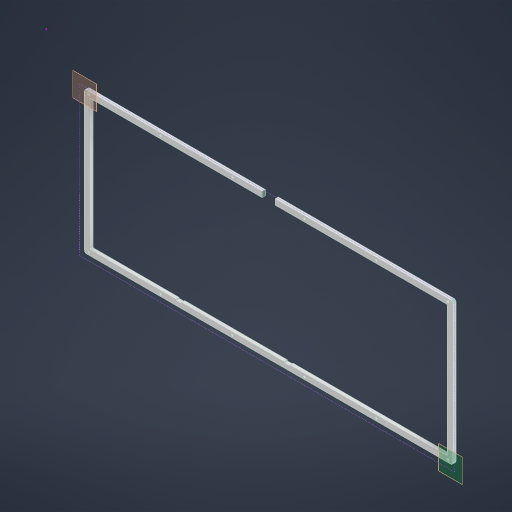
# Autodesk Inventor part: closed_liner
Saved by Autodesk Inventor 2024.2 (Build 282272000, 272)
## iProperties
Created: 2024-06-20
Part Number: closed_liner
Material: Generic
Document SubType Name: Modeling
Designer: Moe
Density: 1 g/cm^3
Appearance: Default
Author: Moe
Autodesk Inventor part; units mm, degrees
ref_plane "YZ Plane" through (0, 0, 0) normal (1, 0, 0) x (0, 1, 0)
ref_plane "XZ Plane" through (0, 0, 0) normal (0, 1, 0) x (-1, 0, 0)
ref_plane "XY Plane" through (0, 0, 0) normal (0, 0, 1) x (1, 0, 0)
ref_plane "Work Plane1" through (35.545, -31.609, 1.6) normal (0, 0, 1) x (1, 0, 0)
sketch "Sketch2" plane through (35.545, -31.609, 1.6) normal (0, 0, 1) x (1, 0, 0)
  line L0 (-4.7778, 3.1171) -> (341.5466, 3.1925) construction
  line L1 (341.5466, 3.1925) -> (341.5765, -133.848) construction
  line L2 (341.5765, -133.848) -> (-4.7479, -133.9235) construction
  line L3 (-4.7479, -133.9235) -> (-4.7778, 3.1171) construction
  point P0 (-35.545, 31.609)
  constraints: 2 other
ref_plane "Work Plane2" through (371.545, -162.609, 0) normal (0, 0, -1) x (-1, 0, 0)
sketch "Sketch8" plane through (371.545, -162.609, 0) normal (0, 0, -1) x (-1, 0, 0)
  line L0 (336, 131) -> (0, 131) projected
  line L1 (-2, 129) -> (-2, 2) projected
  line L2 (-1.9796, 129.2846) -> (-2, 129) projected
  line L3 (-1.919, 129.5635) -> (-1.9796, 129.2846) projected
  line L4 (-0.2846, 130.9796) -> (-0.5635, 130.919) projected
  line L5 (-0.5635, 130.919) -> (-0.8308, 130.8193) projected
  line L6 (-0.8308, 130.8193) -> (-1.0813, 130.6825) projected
  line L7 (-1.0813, 130.6825) -> (-1.3097, 130.5115) projected
  line L8 (-1.3097, 130.5115) -> (-1.5115, 130.3097) projected
  line L9 (-1.5115, 130.3097) -> (-1.6825, 130.0813) projected
  line L10 (-1.6825, 130.0813) -> (-1.8193, 129.8308) projected
  line L11 (-1.8193, 129.8308) -> (-1.919, 129.5635) projected
  line L12 (-1.919, 129.5635) -> (-1.9796, 129.2846) projected
  line L13 (-1.9796, 129.2846) -> (-2, 129) projected
  line L14 (-2, 129) -> (-2, 2) projected
  line L15 (-2, 2) -> (-1.9796, 1.7154) projected
  line L16 (-1.9796, 1.7154) -> (-1.919, 1.4365) projected
  line L17 (-1.919, 1.4365) -> (-1.8193, 1.1692) projected
  line L18 (-1.8193, 1.1692) -> (-1.6825, 0.9187) projected
  line L19 (-1.6825, 0.9187) -> (-1.5115, 0.6903) projected
  line L20 (-1.5115, 0.6903) -> (-1.3097, 0.4885) projected
  line L21 (-1.3097, 0.4885) -> (-1.0813, 0.3175) projected
  line L22 (-1.0813, 0.3175) -> (-0.8308, 0.1807) projected
  line L23 (-0.8308, 0.1807) -> (-0.5635, 0.081) projected
  line L24 (-0.5635, 0.081) -> (-0.2846, 0.0204) projected
  line L25 (-0.2846, 0.0204) -> (0, 0) projected
  line L26 (0, 0) -> (336, 0) projected
  line L27 (336, 0) -> (336.2846, 0.0204) projected
  line L28 (336.2846, 0.0204) -> (336.5635, 0.081) projected
  line L29 (336.5635, 0.081) -> (336.8308, 0.1807) projected
  line L30 (336.8308, 0.1807) -> (337.0813, 0.3175) projected
  line L31 (337.0813, 0.3175) -> (337.3097, 0.4885) projected
  line L32 (337.3097, 0.4885) -> (337.5115, 0.6903) projected
  line L33 (337.5115, 0.6903) -> (337.6825, 0.9187) projected
  line L34 (337.6825, 0.9187) -> (337.8193, 1.1692) projected
  line L35 (337.8193, 1.1692) -> (337.919, 1.4365) projected
  line L36 (337.919, 1.4365) -> (337.9796, 1.7154) projected
  line L37 (337.9796, 1.7154) -> (338, 2) projected
  line L38 (338, 2) -> (338, 129) projected
  line L39 (338, 129) -> (337.9796, 129.2846) projected
  line L40 (337.9796, 129.2846) -> (337.919, 129.5635) projected
  line L41 (337.919, 129.5635) -> (337.8193, 129.8308) projected
  line L42 (337.8193, 129.8308) -> (337.6825, 130.0813) projected
  line L43 (337.6825, 130.0813) -> (337.5115, 130.3097) projected
  line L44 (337.5115, 130.3097) -> (337.3097, 130.5115) projected
  line L45 (337.3097, 130.5115) -> (337.0813, 130.6825) projected
  line L46 (337.0813, 130.6825) -> (336.8308, 130.8193) projected
  line L47 (336.8308, 130.8193) -> (336.5635, 130.919) projected
  line L48 (336.5635, 130.919) -> (336.2846, 130.9796) projected
  line L49 (336.2846, 130.9796) -> (336, 131) projected
  line L50 (336, 131) -> (0, 131) projected
  line L51 (0, 131) -> (-0.2846, 130.9796) projected
  circle A0 centre (2.355, 2.37) radius 1.1 projected
  circle A1 centre (25.63, 14.018) radius 0.875 projected
  circle A2 centre (30.71, 14.018) radius 1.9939 projected
  circle A3 centre (35.79, 14.018) radius 0.875 projected
  circle A4 centre (34.52, 16.558) radius 1.5 projected
  circle A5 centre (68.688, 2.37) radius 1.1 projected
  circle A6 centre (44.68, 14.018) radius 0.875 projected
  circle A7 centre (49.76, 14.018) radius 1.9939 projected
  circle A8 centre (54.84, 14.018) radius 0.875 projected
  circle A9 centre (63.73, 14.018) radius 0.875 projected
  circle A10 centre (53.57, 16.558) radius 1.5 projected
  circle A11 centre (68.81, 14.018) radius 1.9939 projected
  circle A12 centre (73.89, 14.018) radius 0.875 projected
  circle A13 centre (72.62, 16.558) radius 1.5 projected
  circle A14 centre (28.17, 19.098) radius 1.5 projected
  circle A15 centre (47.22, 19.098) radius 1.5 projected
  circle A16 centre (66.27, 19.098) radius 1.5 projected
  circle A17 centre (44.68, 33.068) radius 0.875 projected
  circle A18 centre (49.76, 33.068) radius 1.9939 projected
  circle A19 centre (54.84, 33.068) radius 0.875 projected
  circle A20 centre (88.7635, 15.507) radius 0.875 projected
  circle A21 centre (93.8435, 15.507) radius 1.9939 projected
  circle A22 centre (98.9235, 15.507) radius 0.875 projected
  circle A23 centre (107.8135, 15.507) radius 0.875 projected
  circle A24 centre (112.8935, 15.507) radius 1.9939 projected
  circle A25 centre (117.9735, 15.507) radius 0.875 projected
  circle A26 centre (135.021, 2.37) radius 1.1 projected
  circle A27 centre (150.9996, 7.252) radius 1.9939 projected
  circle A28 centre (126.8635, 15.507) radius 0.875 projected
  circle A29 centre (131.9435, 15.507) radius 1.9939 projected
  circle A30 centre (137.0235, 15.507) radius 0.875 projected
  circle A31 centre (91.3035, 20.587) radius 1.5 projected
  circle A32 centre (97.6535, 18.047) radius 1.5 projected
  circle A33 centre (110.3535, 20.587) radius 1.5 projected
  circle A34 centre (116.7035, 18.047) radius 1.5 projected
  circle A35 centre (135.7535, 18.047) radius 1.5 projected
  circle A36 centre (129.4035, 20.587) radius 1.5 projected
  circle A37 centre (150.9996, 22.492) radius 1.524 projected
  circle A38 centre (15.263, 34.033) radius 0.175 projected
  circle A39 centre (16.538, 34.033) radius 0.175 projected
  circle A40 centre (15.263, 35.308) radius 0.175 projected
  circle A41 centre (16.538, 35.308) radius 0.175 projected
  circle A42 centre (17.813, 34.033) radius 0.175 projected
  circle A43 centre (17.813, 35.308) radius 0.175 projected
  circle A44 centre (15.263, 36.583) radius 0.175 projected
  circle A45 centre (16.538, 36.583) radius 0.175 projected
  circle A46 centre (17.813, 36.583) radius 0.175 projected
  circle A47 centre (53.57, 35.608) radius 1.5 projected
  circle A48 centre (47.22, 38.148) radius 1.5 projected
  circle A49 centre (76.8565, 34.557) radius 0.875 projected
  circle A50 centre (81.9365, 34.557) radius 1.9939 projected
  circle A51 centre (79.3965, 39.637) radius 1.5 projected
  circle A52 centre (55.7115, 45.352) radius 1.9939 projected
  circle A53 centre (79.5875, 45.352) radius 1.9939 projected
  circle A54 centre (40.503, 50.621) radius 0.5 projected
  circle A55 centre (40.503, 53.161) radius 0.5 projected
  circle A56 centre (40.503, 55.701) radius 0.5 projected
  circle A57 centre (40.503, 58.241) radius 0.5 projected
  circle A58 centre (62.5695, 53.607) radius 0.875 projected
  circle A59 centre (67.6495, 53.607) radius 1.9939 projected
  circle A60 centre (72.7295, 53.607) radius 0.875 projected
  circle A61 centre (71.4595, 56.147) radius 1.5 projected
  circle A62 centre (55.7115, 60.592) radius 1.524 projected
  circle A63 centre (65.1095, 58.687) radius 1.5 projected
  circle A64 centre (79.5875, 60.592) radius 1.524 projected
  circle A65 centre (87.0165, 34.557) radius 0.875 projected
  circle A66 centre (85.7465, 37.097) radius 1.5 projected
  circle A67 centre (103.0505, 34.557) radius 0.875 projected
  circle A68 centre (108.1305, 34.557) radius 1.9939 projected
  circle A69 centre (113.2105, 34.557) radius 0.875 projected
  circle A70 centre (111.9405, 37.097) radius 1.5 projected
  circle A71 centre (122.1005, 34.557) radius 0.875 projected
  circle A72 centre (105.5905, 39.637) radius 1.5 projected
  circle A73 centre (124.6405, 39.637) radius 1.5 projected
  circle A74 centre (127.1805, 34.557) radius 1.9939 projected
  circle A75 centre (132.2605, 34.557) radius 0.875 projected
  circle A76 centre (130.9905, 37.097) radius 1.5 projected
  circle A77 centre (141.1505, 34.557) radius 0.875 projected
  circle A78 centre (146.2305, 34.557) radius 1.9939 projected
  circle A79 centre (143.6905, 39.637) radius 1.5 projected
  circle A80 centre (151.3105, 34.557) radius 0.875 projected
  circle A81 centre (150.0405, 37.097) radius 1.5 projected
  circle A82 centre (160.2005, 34.557) radius 0.875 projected
  circle A83 centre (165.2805, 34.557) radius 1.9939 projected
  circle A84 centre (162.7405, 39.637) radius 1.5 projected
  circle A85 centre (93.5255, 53.607) radius 0.875 projected
  circle A86 centre (98.6055, 53.607) radius 1.9939 projected
  circle A87 centre (103.6855, 53.607) radius 0.875 projected
  circle A88 centre (102.4155, 56.147) radius 1.5 projected
  circle A89 centre (112.5755, 53.607) radius 0.875 projected
  circle A90 centre (117.6555, 53.607) radius 1.9939 projected
  circle A91 centre (122.7355, 53.607) radius 0.875 projected
  circle A92 centre (121.4655, 56.147) radius 1.5 projected
  circle A93 centre (96.0655, 58.687) radius 1.5 projected
  circle A94 centre (115.1155, 58.687) radius 1.5 projected
  circle A95 centre (131.6255, 53.607) radius 0.875 projected
  circle A96 centre (136.7055, 53.607) radius 1.9939 projected
  circle A97 centre (141.7855, 53.607) radius 0.875 projected
  circle A98 centre (140.5155, 56.147) radius 1.5 projected
  circle A99 centre (150.6755, 53.607) radius 0.875 projected
  circle A100 centre (155.7555, 53.607) radius 1.9939 projected
  circle A101 centre (160.8355, 53.607) radius 0.875 projected
  circle A102 centre (159.5655, 56.147) radius 1.5 projected
  circle A103 centre (134.1655, 58.687) radius 1.5 projected
  circle A104 centre (153.2155, 58.687) radius 1.5 projected
  circle A105 centre (201.354, 2.37) radius 1.1 projected
  circle A106 centre (195.9195, 15.507) radius 0.875 projected
  circle A107 centre (200.9995, 15.507) radius 1.9939 projected
  circle A108 centre (206.0795, 15.507) radius 0.875 projected
  circle A109 centre (250.9994, 7.252) radius 1.9939 projected
  circle A110 centre (198.4595, 20.587) radius 1.5 projected
  circle A111 centre (204.8095, 18.047) radius 1.5 projected
  circle A112 centre (250.9994, 22.492) radius 1.524 projected
  circle A113 centre (267.687, 2.37) radius 1.1 projected
  circle A114 centre (267.3575, 15.507) radius 0.875 projected
  circle A115 centre (272.4375, 15.507) radius 1.9939 projected
  circle A116 centre (277.5175, 15.507) radius 0.875 projected
  circle A117 centre (291.1705, 15.507) radius 0.875 projected
  circle A118 centre (334.02, 2.37) radius 1.1 projected
  circle A119 centre (296.2505, 15.507) radius 1.9939 projected
  circle A120 centre (301.3305, 15.507) radius 0.875 projected
  circle A121 centre (314.9835, 15.507) radius 0.875 projected
  circle A122 centre (320.0635, 15.507) radius 1.9939 projected
  circle A123 centre (325.1435, 15.507) radius 0.875 projected
  circle A124 centre (269.8975, 20.587) radius 1.5 projected
  circle A125 centre (276.2475, 18.047) radius 1.5 projected
  circle A126 centre (300.0605, 18.047) radius 1.5 projected
  circle A127 centre (293.7105, 20.587) radius 1.5 projected
  circle A128 centre (323.8735, 18.047) radius 1.5 projected
  circle A129 centre (317.5235, 20.587) radius 1.5 projected
  circle A130 centre (298.5985, 26.302) radius 1.9939 projected
  circle A131 centre (322.4745, 26.302) radius 1.9939 projected
  circle A132 centre (170.3605, 34.557) radius 0.875 projected
  circle A133 centre (169.0905, 37.097) radius 1.5 projected
  circle A134 centre (179.2505, 34.557) radius 0.875 projected
  circle A135 centre (184.3305, 34.557) radius 1.9939 projected
  circle A136 centre (188.1405, 37.097) radius 1.5 projected
  circle A137 centre (181.7905, 39.637) radius 1.5 projected
  circle A138 centre (189.4105, 34.557) radius 0.875 projected
  circle A139 centre (198.3005, 34.557) radius 0.875 projected
  circle A140 centre (203.3805, 34.557) radius 1.9939 projected
  circle A141 centre (208.4605, 34.557) radius 0.875 projected
  circle A142 centre (207.1905, 37.097) radius 1.5 projected
  circle A143 centre (200.8405, 39.637) radius 1.5 projected
  circle A144 centre (217.3505, 34.557) radius 0.875 projected
  circle A145 centre (222.4305, 34.557) radius 1.9939 projected
  circle A146 centre (227.5105, 34.557) radius 0.875 projected
  circle A147 centre (226.2405, 37.097) radius 1.5 projected
  circle A148 centre (219.8905, 39.637) radius 1.5 projected
  circle A149 centre (236.4005, 34.557) radius 0.875 projected
  circle A150 centre (241.4805, 34.557) radius 1.9939 projected
  circle A151 centre (246.5605, 34.557) radius 0.875 projected
  circle A152 centre (245.2905, 37.097) radius 1.5 projected
  circle A153 centre (238.9405, 39.637) radius 1.5 projected
  circle A154 centre (169.7255, 53.607) radius 0.875 projected
  circle A155 centre (174.8055, 53.607) radius 1.9939 projected
  circle A156 centre (179.8855, 53.607) radius 0.875 projected
  circle A157 centre (188.7755, 53.607) radius 0.875 projected
  circle A158 centre (178.6155, 56.147) radius 1.5 projected
  circle A159 centre (193.8555, 53.607) radius 1.9939 projected
  circle A160 centre (198.9355, 53.607) radius 0.875 projected
  circle A161 centre (207.8255, 53.607) radius 0.875 projected
  circle A162 centre (197.6655, 56.147) radius 1.5 projected
  circle A163 centre (172.2655, 58.687) radius 1.5 projected
  circle A164 centre (191.3155, 58.687) radius 1.5 projected
  circle A165 centre (212.9055, 53.607) radius 1.9939 projected
  circle A166 centre (217.9855, 53.607) radius 0.875 projected
  circle A167 centre (226.8755, 53.607) radius 0.875 projected
  circle A168 centre (216.7155, 56.147) radius 1.5 projected
  circle A169 centre (231.9555, 53.607) radius 1.9939 projected
  circle A170 centre (237.0355, 53.607) radius 0.875 projected
  circle A171 centre (245.9255, 53.607) radius 0.875 projected
  circle A172 centre (251.0055, 53.607) radius 1.9939 projected
  circle A173 centre (235.7655, 56.147) radius 1.5 projected
  circle A174 centre (210.3655, 58.687) radius 1.5 projected
  circle A175 centre (229.4155, 58.687) radius 1.5 projected
  circle A176 centre (248.4655, 58.687) radius 1.5 projected
  circle A177 centre (255.4505, 34.557) radius 0.875 projected
  circle A178 centre (260.5305, 34.557) radius 1.9939 projected
  circle A179 centre (265.6105, 34.557) radius 0.875 projected
  circle A180 centre (264.3405, 37.097) radius 1.5 projected
  circle A181 centre (257.9905, 39.637) radius 1.5 projected
  circle A182 centre (274.5005, 34.557) radius 0.875 projected
  circle A183 centre (279.5805, 34.557) radius 1.9939 projected
  circle A184 centre (284.6605, 34.557) radius 0.875 projected
  circle A185 centre (283.3905, 37.097) radius 1.5 projected
  circle A186 centre (277.0405, 39.637) radius 1.5 projected
  circle A187 centre (305.4565, 34.557) radius 0.875 projected
  circle A188 centre (310.5365, 34.557) radius 1.9939 projected
  circle A189 centre (298.5985, 41.542) radius 1.524 projected
  circle A190 centre (307.9965, 39.637) radius 1.5 projected
  circle A191 centre (315.6165, 34.557) radius 0.875 projected
  circle A192 centre (314.3465, 37.097) radius 1.5 projected
  circle A193 centre (322.4745, 41.542) radius 1.524 projected
  circle A194 centre (256.0855, 53.607) radius 0.875 projected
  circle A195 centre (264.9755, 53.607) radius 0.875 projected
  circle A196 centre (270.0555, 53.607) radius 1.9939 projected
  circle A197 centre (254.8155, 56.147) radius 1.5 projected
  circle A198 centre (275.1355, 53.607) radius 0.875 projected
  circle A199 centre (284.0255, 53.607) radius 0.875 projected
  circle A200 centre (289.1055, 53.607) radius 1.9939 projected
  circle A201 centre (273.8655, 56.147) radius 1.5 projected
  circle A202 centre (292.9155, 56.147) radius 1.5 projected
  circle A203 centre (267.5155, 58.687) radius 1.5 projected
  circle A204 centre (286.5655, 58.687) radius 1.5 projected
  circle A205 centre (294.1855, 53.607) radius 0.875 projected
  circle A206 centre (310.2195, 53.607) radius 0.875 projected
  circle A207 centre (315.2995, 53.607) radius 1.9939 projected
  circle A208 centre (320.3795, 53.607) radius 0.875 projected
  circle A209 centre (319.1095, 56.147) radius 1.5 projected
  circle A210 centre (312.7595, 58.687) radius 1.5 projected
  circle A211 centre (8.119, 72.666) radius 0.875 projected
  circle A212 centre (13.199, 72.666) radius 1.9939 projected
  circle A213 centre (18.279, 72.666) radius 0.875 projected
  circle A214 centre (27.169, 72.666) radius 0.875 projected
  circle A215 centre (32.249, 72.666) radius 1.9939 projected
  circle A216 centre (37.329, 72.666) radius 0.875 projected
  circle A217 centre (10.659, 77.746) radius 1.5 projected
  circle A218 centre (17.009, 75.206) radius 1.5 projected
  circle A219 centre (29.709, 77.746) radius 1.5 projected
  circle A220 centre (36.059, 75.206) radius 1.5 projected
  circle A221 centre (55.4245, 72.657) radius 0.875 projected
  circle A222 centre (60.5045, 72.657) radius 1.9939 projected
  circle A223 centre (65.5845, 72.657) radius 0.875 projected
  circle A224 centre (79.2375, 72.657) radius 0.875 projected
  circle A225 centre (84.3175, 72.657) radius 1.9939 projected
  circle A226 centre (57.9645, 77.737) radius 1.5 projected
  circle A227 centre (64.3145, 75.197) radius 1.5 projected
  circle A228 centre (81.7775, 77.737) radius 1.5 projected
  circle A229 centre (8.119, 91.716) radius 0.875 projected
  circle A230 centre (13.199, 91.716) radius 1.9939 projected
  circle A231 centre (18.279, 91.716) radius 0.875 projected
  circle A232 centre (10.659, 96.796) radius 1.5 projected
  circle A233 centre (17.009, 94.256) radius 1.5 projected
  circle A234 centre (27.169, 91.716) radius 0.875 projected
  circle A235 centre (32.249, 91.716) radius 1.9939 projected
  circle A236 centre (37.329, 91.716) radius 0.875 projected
  circle A237 centre (29.709, 96.796) radius 1.5 projected
  circle A238 centre (36.059, 94.256) radius 1.5 projected
  circle A239 centre (53.33, 83.452) radius 1.9939 projected
  circle A240 centre (77.206, 83.452) radius 1.9939 projected
  circle A241 centre (60.188, 91.707) radius 0.875 projected
  circle A242 centre (62.728, 96.787) radius 1.5 projected
  circle A243 centre (65.268, 91.707) radius 1.9939 projected
  circle A244 centre (70.348, 91.707) radius 0.875 projected
  circle A245 centre (69.078, 94.247) radius 1.5 projected
  circle A246 centre (89.3975, 72.657) radius 0.875 projected
  circle A247 centre (98.2875, 72.657) radius 0.875 projected
  circle A248 centre (103.3675, 72.657) radius 1.9939 projected
  circle A249 centre (108.4475, 72.657) radius 0.875 projected
  circle A250 centre (117.3375, 72.657) radius 0.875 projected
  circle A251 centre (122.4175, 72.657) radius 1.9939 projected
  circle A252 centre (88.1275, 75.197) radius 1.5 projected
  circle A253 centre (100.8275, 77.737) radius 1.5 projected
  circle A254 centre (107.1775, 75.197) radius 1.5 projected
  circle A255 centre (126.2275, 75.197) radius 1.5 projected
  circle A256 centre (119.8775, 77.737) radius 1.5 projected
  circle A257 centre (127.4975, 72.657) radius 0.875 projected
  circle A258 centre (136.3875, 72.657) radius 0.875 projected
  circle A259 centre (141.4675, 72.657) radius 1.9939 projected
  circle A260 centre (146.5475, 72.657) radius 0.875 projected
  circle A261 centre (155.4375, 72.657) radius 0.875 projected
  circle A262 centre (160.5175, 72.657) radius 1.9939 projected
  circle A263 centre (165.5975, 72.657) radius 0.875 projected
  circle A264 centre (145.2775, 75.197) radius 1.5 projected
  circle A265 centre (138.9275, 77.737) radius 1.5 projected
  circle A266 centre (164.3275, 75.197) radius 1.5 projected
  circle A267 centre (157.9775, 77.737) radius 1.5 projected
  circle A268 centre (88.763, 91.707) radius 0.875 projected
  circle A269 centre (93.843, 91.707) radius 1.9939 projected
  circle A270 centre (98.923, 91.707) radius 0.875 projected
  circle A271 centre (91.303, 96.787) radius 1.5 projected
  circle A272 centre (97.653, 94.247) radius 1.5 projected
  circle A273 centre (107.813, 91.707) radius 0.875 projected
  circle A274 centre (112.893, 91.707) radius 1.9939 projected
  circle A275 centre (117.973, 91.707) radius 0.875 projected
  circle A276 centre (110.353, 96.787) radius 1.5 projected
  circle A277 centre (116.703, 94.247) radius 1.5 projected
  circle A278 centre (126.863, 91.707) radius 0.875 projected
  circle A279 centre (131.943, 91.707) radius 1.9939 projected
  circle A280 centre (137.023, 91.707) radius 0.875 projected
  circle A281 centre (145.913, 91.707) radius 0.875 projected
  circle A282 centre (135.753, 94.247) radius 1.5 projected
  circle A283 centre (129.403, 96.787) radius 1.5 projected
  circle A284 centre (150.993, 91.707) radius 1.9939 projected
  circle A285 centre (156.073, 91.707) radius 0.875 projected
  circle A286 centre (164.963, 91.707) radius 0.875 projected
  circle A287 centre (154.803, 94.247) radius 1.5 projected
  circle A288 centre (148.453, 96.787) radius 1.5 projected
  circle A289 centre (167.503, 96.787) radius 1.5 projected
  circle A290 centre (41.979, 103.44) radius 1.1 projected
  circle A291 centre (16.298, 112.417) radius 0.5 projected
  circle A292 centre (23.298, 109.317) radius 1.3 projected
  circle A293 centre (30.798, 112.417) radius 0.5 projected
  circle A294 centre (53.33, 98.692) radius 1.524 projected
  circle A295 centre (77.206, 98.692) radius 1.524 projected
  circle A296 centre (16.298, 117.417) radius 0.5 projected
  circle A297 centre (30.798, 114.917) radius 0.5 projected
  circle A298 centre (30.798, 117.417) radius 0.5 projected
  circle A299 centre (23.298, 120.517) radius 1.3 projected
  circle A300 centre (2.362, 128.645) radius 1.1 projected
  circle A301 centre (50.683, 115.519) radius 0.875 projected
  circle A302 centre (55.763, 115.519) radius 1.9939 projected
  circle A303 centre (60.843, 115.519) radius 0.875 projected
  circle A304 centre (59.573, 118.059) radius 1.5 projected
  circle A305 centre (53.223, 120.599) radius 1.5 projected
  circle A306 centre (76.277, 115.499) radius 0.875 projected
  circle A307 centre (81.357, 115.499) radius 1.9939 projected
  circle A308 centre (78.817, 120.579) radius 1.5 projected
  circle A309 centre (68.695, 128.645) radius 1.1 projected
  circle A310 centre (125.979, 103.44) radius 1.1 projected
  circle A311 centre (86.437, 115.499) radius 0.875 projected
  circle A312 centre (85.167, 118.039) radius 1.5 projected
  circle A313 centre (95.327, 115.499) radius 0.875 projected
  circle A314 centre (100.407, 115.499) radius 1.9939 projected
  circle A315 centre (105.487, 115.499) radius 0.875 projected
  circle A316 centre (104.217, 118.039) radius 1.5 projected
  circle A317 centre (97.867, 120.579) radius 1.5 projected
  circle A318 centre (114.377, 115.499) radius 0.875 projected
  circle A319 centre (119.457, 115.499) radius 1.9939 projected
  circle A320 centre (124.537, 115.499) radius 0.875 projected
  circle A321 centre (123.267, 118.039) radius 1.5 projected
  circle A322 centre (116.917, 120.579) radius 1.5 projected
  circle A323 centre (133.427, 115.499) radius 0.875 projected
  circle A324 centre (138.507, 115.499) radius 1.9939 projected
  circle A325 centre (143.587, 115.499) radius 0.875 projected
  circle A326 centre (142.317, 118.039) radius 1.5 projected
  circle A327 centre (135.967, 120.579) radius 1.5 projected
  circle A328 centre (156.652, 115.499) radius 0.875 projected
  circle A329 centre (161.732, 115.499) radius 1.9939 projected
  circle A330 centre (166.812, 115.499) radius 0.875 projected
  circle A331 centre (165.542, 118.039) radius 1.5 projected
  circle A332 centre (159.192, 120.579) radius 1.5 projected
  circle A333 centre (135.028, 128.645) radius 1.1 projected
  line L52 (163.9729, 126.3401) -> (163.9331, 126.4429) projected
  line L53 (163.978, 126.285) -> (163.9729, 126.3401) projected
  line L54 (163.978, 125.185) -> (163.978, 126.285) projected
  line L55 (163.9577, 125.0766) -> (163.978, 125.185) projected
  line L56 (163.8997, 124.9829) -> (163.9577, 125.0766) projected
  line L57 (163.8117, 124.9165) -> (163.8997, 124.9829) projected
  line L58 (163.7057, 124.8863) -> (163.8117, 124.9165) projected
  line L59 (163.5959, 124.8965) -> (163.7057, 124.8863) projected
  line L60 (163.4972, 124.9456) -> (163.5959, 124.8965) projected
  line L61 (163.4229, 125.0271) -> (163.4972, 124.9456) projected
  line L62 (163.3831, 125.1299) -> (163.4229, 125.0271) projected
  line L63 (163.378, 125.185) -> (163.3831, 125.1299) projected
  line L64 (163.378, 126.285) -> (163.378, 125.185) projected
  line L65 (163.3983, 126.3934) -> (163.378, 126.285) projected
  line L66 (163.4563, 126.4871) -> (163.3983, 126.3934) projected
  line L67 (163.5443, 126.5535) -> (163.4563, 126.4871) projected
  line L68 (163.6503, 126.5837) -> (163.5443, 126.5535) projected
  line L69 (163.7601, 126.5735) -> (163.6503, 126.5837) projected
  line L70 (163.8588, 126.5244) -> (163.7601, 126.5735) projected
  line L71 (163.9331, 126.4429) -> (163.8588, 126.5244) projected
  circle A334 centre (165.108, 126.265) radius 0.325 projected
  line L72 (163.9729, 130.2701) -> (163.9331, 130.3729) projected
  line L73 (163.978, 130.215) -> (163.9729, 130.2701) projected
  line L74 (163.978, 129.615) -> (163.978, 130.215) projected
  line L75 (163.9577, 129.5066) -> (163.978, 129.615) projected
  line L76 (163.8997, 129.4129) -> (163.9577, 129.5066) projected
  line L77 (163.8117, 129.3465) -> (163.8997, 129.4129) projected
  line L78 (163.7057, 129.3163) -> (163.8117, 129.3465) projected
  line L79 (163.5959, 129.3265) -> (163.7057, 129.3163) projected
  line L80 (163.4972, 129.3756) -> (163.5959, 129.3265) projected
  line L81 (163.4229, 129.4571) -> (163.4972, 129.3756) projected
  line L82 (163.3831, 129.5599) -> (163.4229, 129.4571) projected
  line L83 (163.378, 129.615) -> (163.3831, 129.5599) projected
  line L84 (163.378, 130.215) -> (163.378, 129.615) projected
  line L85 (163.3983, 130.3234) -> (163.378, 130.215) projected
  line L86 (163.4563, 130.4171) -> (163.3983, 130.3234) projected
  line L87 (163.5443, 130.4835) -> (163.4563, 130.4171) projected
  line L88 (163.6503, 130.5137) -> (163.5443, 130.4835) projected
  line L89 (163.7601, 130.5035) -> (163.6503, 130.5137) projected
  line L90 (163.8588, 130.4544) -> (163.7601, 130.5035) projected
  line L91 (163.9331, 130.3729) -> (163.8588, 130.4544) projected
  circle A335 centre (174.4875, 72.657) radius 0.875 projected
  circle A336 centre (179.5675, 72.657) radius 1.9939 projected
  circle A337 centre (184.6475, 72.657) radius 0.875 projected
  circle A338 centre (193.5375, 72.657) radius 0.875 projected
  circle A339 centre (198.6175, 72.657) radius 1.9939 projected
  circle A340 centre (203.6975, 72.657) radius 0.875 projected
  circle A341 centre (177.0275, 77.737) radius 1.5 projected
  circle A342 centre (183.3775, 75.197) radius 1.5 projected
  circle A343 centre (196.0775, 77.737) radius 1.5 projected
  circle A344 centre (202.4275, 75.197) radius 1.5 projected
  circle A345 centre (212.5875, 72.657) radius 0.875 projected
  circle A346 centre (217.6675, 72.657) radius 1.9939 projected
  circle A347 centre (222.7475, 72.657) radius 0.875 projected
  circle A348 centre (231.6375, 72.657) radius 0.875 projected
  circle A349 centre (236.7175, 72.657) radius 1.9939 projected
  circle A350 centre (241.7975, 72.657) radius 0.875 projected
  circle A351 centre (250.6875, 72.657) radius 0.875 projected
  circle A352 centre (215.1275, 77.737) radius 1.5 projected
  circle A353 centre (221.4775, 75.197) radius 1.5 projected
  circle A354 centre (240.5275, 75.197) radius 1.5 projected
  circle A355 centre (234.1775, 77.737) radius 1.5 projected
  circle A356 centre (170.043, 91.707) radius 1.9939 projected
  circle A357 centre (175.123, 91.707) radius 0.875 projected
  circle A358 centre (184.013, 91.707) radius 0.875 projected
  circle A359 centre (173.853, 94.247) radius 1.5 projected
  circle A360 centre (186.553, 96.787) radius 1.5 projected
  circle A361 centre (189.093, 91.707) radius 1.9939 projected
  circle A362 centre (194.173, 91.707) radius 0.875 projected
  circle A363 centre (203.063, 91.707) radius 0.875 projected
  circle A364 centre (208.143, 91.707) radius 1.9939 projected
  circle A365 centre (192.903, 94.247) radius 1.5 projected
  circle A366 centre (205.603, 96.787) radius 1.5 projected
  circle A367 centre (213.223, 91.707) radius 0.875 projected
  circle A368 centre (222.113, 91.707) radius 0.875 projected
  circle A369 centre (227.193, 91.707) radius 1.9939 projected
  circle A370 centre (211.953, 94.247) radius 1.5 projected
  circle A371 centre (224.653, 96.787) radius 1.5 projected
  circle A372 centre (232.273, 91.707) radius 0.875 projected
  circle A373 centre (241.163, 91.707) radius 0.875 projected
  circle A374 centre (246.243, 91.707) radius 1.9939 projected
  circle A375 centre (251.323, 91.707) radius 0.875 projected
  circle A376 centre (231.003, 94.247) radius 1.5 projected
  circle A377 centre (250.053, 94.247) radius 1.5 projected
  circle A378 centre (243.703, 96.787) radius 1.5 projected
  circle A379 centre (255.7675, 72.657) radius 1.9939 projected
  circle A380 centre (260.8475, 72.657) radius 0.875 projected
  circle A381 centre (269.7375, 72.657) radius 0.875 projected
  circle A382 centre (274.8175, 72.657) radius 1.9939 projected
  circle A383 centre (279.8975, 72.657) radius 0.875 projected
  circle A384 centre (288.7875, 72.657) radius 0.875 projected
  circle A385 centre (259.5775, 75.197) radius 1.5 projected
  circle A386 centre (253.2275, 77.737) radius 1.5 projected
  circle A387 centre (272.2775, 77.737) radius 1.5 projected
  circle A388 centre (278.6275, 75.197) radius 1.5 projected
  circle A389 centre (291.3275, 77.737) radius 1.5 projected
  circle A390 centre (293.8675, 72.657) radius 1.9939 projected
  circle A391 centre (298.9475, 72.657) radius 0.875 projected
  circle A392 centre (312.6005, 72.657) radius 0.875 projected
  circle A393 centre (317.6805, 72.657) radius 1.9939 projected
  circle A394 centre (322.7605, 72.657) radius 0.875 projected
  circle A395 centre (297.6775, 75.197) radius 1.5 projected
  circle A396 centre (321.4905, 75.197) radius 1.5 projected
  circle A397 centre (315.1405, 77.737) radius 1.5 projected
  circle A398 centre (260.213, 91.707) radius 0.875 projected
  circle A399 centre (265.293, 91.707) radius 1.9939 projected
  circle A400 centre (270.373, 91.707) radius 0.875 projected
  circle A401 centre (269.103, 94.247) radius 1.5 projected
  circle A402 centre (262.753, 96.787) radius 1.5 projected
  circle A403 centre (279.263, 91.707) radius 0.875 projected
  circle A404 centre (284.343, 91.707) radius 1.9939 projected
  circle A405 centre (289.423, 91.707) radius 0.875 projected
  circle A406 centre (281.803, 96.787) radius 1.5 projected
  circle A407 centre (288.153, 94.247) radius 1.5 projected
  circle A408 centre (298.313, 91.707) radius 0.875 projected
  circle A409 centre (303.393, 91.707) radius 1.9939 projected
  circle A410 centre (308.473, 91.707) radius 0.875 projected
  circle A411 centre (300.853, 96.787) radius 1.5 projected
  circle A412 centre (307.203, 94.247) radius 1.5 projected
  circle A413 centre (317.363, 91.707) radius 0.875 projected
  circle A414 centre (322.443, 91.707) radius 1.9939 projected
  circle A415 centre (327.523, 91.707) radius 0.875 projected
  circle A416 centre (319.903, 96.787) radius 1.5 projected
  circle A417 centre (326.253, 94.247) radius 1.5 projected
  circle A418 centre (210.039, 103.527) radius 1.1 projected
  circle A419 centre (175.702, 115.499) radius 0.875 projected
  circle A420 centre (180.782, 115.499) radius 1.9939 projected
  circle A421 centre (185.862, 115.499) radius 0.875 projected
  circle A422 centre (184.592, 118.039) radius 1.5 projected
  circle A423 centre (178.242, 120.579) radius 1.5 projected
  circle A424 centre (194.752, 115.499) radius 0.875 projected
  circle A425 centre (199.832, 115.499) radius 1.9939 projected
  circle A426 centre (204.912, 115.499) radius 0.875 projected
  circle A427 centre (203.642, 118.039) radius 1.5 projected
  circle A428 centre (197.292, 120.579) radius 1.5 projected
  line L92 (172.6129, 126.3401) -> (172.5731, 126.4429) projected
  line L93 (172.618, 126.285) -> (172.6129, 126.3401) projected
  line L94 (172.618, 125.185) -> (172.618, 126.285) projected
  line L95 (172.5977, 125.0766) -> (172.618, 125.185) projected
  line L96 (172.5397, 124.9829) -> (172.5977, 125.0766) projected
  line L97 (172.4517, 124.9165) -> (172.5397, 124.9829) projected
  line L98 (172.3457, 124.8863) -> (172.4517, 124.9165) projected
  line L99 (172.2359, 124.8965) -> (172.3457, 124.8863) projected
  line L100 (172.1372, 124.9456) -> (172.2359, 124.8965) projected
  line L101 (172.0629, 125.0271) -> (172.1372, 124.9456) projected
  line L102 (172.0231, 125.1299) -> (172.0629, 125.0271) projected
  line L103 (172.018, 125.185) -> (172.0231, 125.1299) projected
  line L104 (172.018, 126.285) -> (172.018, 125.185) projected
  line L105 (172.0383, 126.3934) -> (172.018, 126.285) projected
  line L106 (172.0963, 126.4871) -> (172.0383, 126.3934) projected
  line L107 (172.1843, 126.5535) -> (172.0963, 126.4871) projected
  line L108 (172.2903, 126.5837) -> (172.1843, 126.5535) projected
  line L109 (172.4001, 126.5735) -> (172.2903, 126.5837) projected
  line L110 (172.4988, 126.5244) -> (172.4001, 126.5735) projected
  line L111 (172.5731, 126.4429) -> (172.4988, 126.5244) projected
  circle A429 centre (170.888, 126.265) radius 0.325 projected
  line L112 (172.6129, 130.2701) -> (172.5731, 130.3729) projected
  line L113 (172.618, 130.215) -> (172.6129, 130.2701) projected
  line L114 (172.618, 129.615) -> (172.618, 130.215) projected
  line L115 (172.5977, 129.5066) -> (172.618, 129.615) projected
  line L116 (172.5397, 129.4129) -> (172.5977, 129.5066) projected
  line L117 (172.4517, 129.3465) -> (172.5397, 129.4129) projected
  line L118 (172.3457, 129.3163) -> (172.4517, 129.3465) projected
  line L119 (172.2359, 129.3265) -> (172.3457, 129.3163) projected
  line L120 (172.1372, 129.3756) -> (172.2359, 129.3265) projected
  line L121 (172.0629, 129.4571) -> (172.1372, 129.3756) projected
  line L122 (172.0231, 129.5599) -> (172.0629, 129.4571) projected
  line L123 (172.018, 129.615) -> (172.0231, 129.5599) projected
  line L124 (172.018, 130.215) -> (172.018, 129.615) projected
  line L125 (172.0383, 130.3234) -> (172.018, 130.215) projected
  line L126 (172.0963, 130.4171) -> (172.0383, 130.3234) projected
  line L127 (172.1843, 130.4835) -> (172.0963, 130.4171) projected
  line L128 (172.2903, 130.5137) -> (172.1843, 130.4835) projected
  line L129 (172.4001, 130.5035) -> (172.2903, 130.5137) projected
  line L130 (172.4988, 130.4544) -> (172.4001, 130.5035) projected
  line L131 (172.5731, 130.3729) -> (172.4988, 130.4544) projected
  circle A430 centre (201.361, 128.645) radius 1.1 projected
  circle A431 centre (213.802, 115.499) radius 0.875 projected
  circle A432 centre (218.882, 115.499) radius 1.9939 projected
  circle A433 centre (223.962, 115.499) radius 0.875 projected
  circle A434 centre (222.692, 118.039) radius 1.5 projected
  circle A435 centre (216.342, 120.579) radius 1.5 projected
  circle A436 centre (237.027, 115.499) radius 0.875 projected
  circle A437 centre (242.107, 115.499) radius 1.9939 projected
  circle A438 centre (247.187, 115.499) radius 0.875 projected
  circle A439 centre (245.917, 118.039) radius 1.5 projected
  circle A440 centre (239.567, 120.579) radius 1.5 projected
  circle A441 centre (294.039, 103.527) radius 1.1 projected
  circle A442 centre (256.077, 115.499) radius 0.875 projected
  circle A443 centre (261.157, 115.499) radius 1.9939 projected
  circle A444 centre (266.237, 115.499) radius 0.875 projected
  circle A445 centre (264.967, 118.039) radius 1.5 projected
  circle A446 centre (258.617, 120.579) radius 1.5 projected
  circle A447 centre (275.127, 115.499) radius 0.875 projected
  circle A448 centre (280.207, 115.499) radius 1.9939 projected
  circle A449 centre (285.287, 115.499) radius 0.875 projected
  circle A450 centre (284.017, 118.039) radius 1.5 projected
  circle A451 centre (277.667, 120.579) radius 1.5 projected
  circle A452 centre (267.694, 128.645) radius 1.1 projected
  circle A453 centre (294.177, 115.499) radius 0.875 projected
  circle A454 centre (299.257, 115.499) radius 1.9939 projected
  circle A455 centre (303.067, 118.039) radius 1.5 projected
  circle A456 centre (304.337, 115.499) radius 0.875 projected
  circle A457 centre (296.717, 120.579) radius 1.5 projected
  circle A458 centre (317.402, 115.477) radius 0.875 projected
  circle A459 centre (322.482, 115.477) radius 1.9939 projected
  circle A460 centre (327.562, 115.477) radius 0.875 projected
  circle A461 centre (326.292, 118.017) radius 1.5 projected
  circle A462 centre (319.942, 120.557) radius 1.5 projected
  circle A463 centre (334.027, 128.645) radius 1.1 projected
  line L132 (4, 126) -> (332, 126)
  line L133 (333, 125) -> (333, 6)
  line L134 (332, 5) -> (4, 5)
  line L135 (3, 6) -> (3, 125)
  arc A464 (333, 125) -> (332, 126) centre (332, 125) ccw
  arc A465 (4, 126) -> (3, 125) centre (4, 125) ccw
  arc A466 (3, 6) -> (4, 5) centre (4, 6) ccw
  arc A467 (332, 5) -> (333, 6) centre (332, 6) ccw
  point P0 (371.545, 162.609)
  point P1 (163.978, 126)
  point P2 (164.9199, 126)
  point P3 (165.2961, 126)
  point P4 (170.6999, 126)
  point P5 (171.0761, 126)
  point P6 (172.018, 126)
  point P7 (172.618, 126)
  point P8 (163.378, 126)
  dimension "d80" = 5
  dimension "d81" = 5
  dimension "d82" = 5
  dimension "d83" = 5
  dimension "d84" = 1
  dimension "d85" = 1
  constraints: 8 end point, 8 point on circle, 8 tangent, 4 centre point, 2 equal radius, 2 parallel, 1 horizontal, 1 perpendicular
  measures "d80" distance between parallel lines of L1 L135
  measures "d81" distance between parallel lines of L0 L132
  measures "d82" distance between parallel lines of L26 L134
  measures "d83" distance between parallel lines of L38 L133
  measures "d84" radius of A464
  measures "d85" radius of A465
extrude "Extrusion3" add sketch "Sketch8" along normal blind 3 contours L49 L48 L47 L46 L45 L44 L43 L42 L41 L40 L39 L38 L37 L36 L35 L34 L33 L32 L31 L30 L29 L28 L27 L26 L25 L24 L23 L22 L21 L20 L19 L18 L17 L16 L15 L1 L2 L3 L11 L10 L9 L8 L7 L6 L5 L4 L51 L0 | L53 L54 L132 L64 L65 L66 L67 L68 L69 L70 L71 L52 | A334 L132 | A429 L132 | L104 L105 L106 L107 L108 L109 L110 L111 L92 L93 L94 L132 | L73 L74 L75 L76 L77 L78 L79 L80 L81 L82 L83 L84 L85 L86 L87 L88 L89 L90 L91 L72 | L113 L114 L115 L116 L117 L118 L119 L120 L121 L122 L123 L124 L125 L126 L127 L128 L129 L130 L131 L112 picked at (165.1275, 126.207) picked at (170.9075, 126.207)
sketch "Sketch9" plane through (371.545, -162.609, -3) normal (0, 0, -1) x (-1, 0, 0)
  line L0 (-2.7439, 132.069) -> (339.0116, 131.9748) construction
  line L1 (339.0116, 131.9748) -> (338.9749, -1.1767) construction
  line L2 (338.9749, -1.1767) -> (-2.7806, -1.0825) construction
  line L3 (-2.7806, -1.0825) -> (-2.7439, 132.069) construction
  circle A0 centre (2.355, 2.37) radius 1.1 projected
  line L4 (-1.919, 129.5635) -> (-1.9796, 129.2846) projected
  line L5 (-1.9796, 129.2846) -> (-2, 129) projected
  line L6 (-2, 129) -> (-2, 2) projected
  line L7 (-2, 2) -> (-1.9796, 1.7154) projected
  line L8 (-1.9796, 1.7154) -> (-1.919, 1.4365) projected
  line L9 (-1.919, 1.4365) -> (-1.8193, 1.1692) projected
  line L10 (-1.8193, 1.1692) -> (-1.6825, 0.9187) projected
  line L11 (-1.6825, 0.9187) -> (-1.5115, 0.6903) projected
  line L12 (-1.5115, 0.6903) -> (-1.3097, 0.4885) projected
  line L13 (-1.3097, 0.4885) -> (-1.0813, 0.3175) projected
  line L14 (-1.0813, 0.3175) -> (-0.8308, 0.1807) projected
  line L15 (-0.8308, 0.1807) -> (-0.5635, 0.081) projected
  line L16 (-0.5635, 0.081) -> (-0.2846, 0.0204) projected
  line L17 (-0.2846, 0.0204) -> (0, 0) projected
  line L18 (0, 0) -> (336, 0) projected
  line L19 (336, 0) -> (336.2846, 0.0204) projected
  line L20 (336.2846, 0.0204) -> (336.5635, 0.081) projected
  line L21 (336.5635, 0.081) -> (336.8308, 0.1807) projected
  line L22 (336.8308, 0.1807) -> (337.0813, 0.3175) projected
  line L23 (337.0813, 0.3175) -> (337.3097, 0.4885) projected
  line L24 (337.3097, 0.4885) -> (337.5115, 0.6903) projected
  line L25 (337.5115, 0.6903) -> (337.6825, 0.9187) projected
  line L26 (337.6825, 0.9187) -> (337.8193, 1.1692) projected
  line L27 (337.8193, 1.1692) -> (337.919, 1.4365) projected
  line L28 (337.919, 1.4365) -> (337.9796, 1.7154) projected
  line L29 (337.9796, 1.7154) -> (338, 2) projected
  line L30 (338, 2) -> (338, 129) projected
  line L31 (338, 129) -> (337.9796, 129.2846) projected
  line L32 (337.9796, 129.2846) -> (337.919, 129.5635) projected
  line L33 (337.919, 129.5635) -> (337.8193, 129.8308) projected
  line L34 (337.8193, 129.8308) -> (337.6825, 130.0813) projected
  line L35 (337.6825, 130.0813) -> (337.5115, 130.3097) projected
  line L36 (337.5115, 130.3097) -> (337.3097, 130.5115) projected
  line L37 (337.3097, 130.5115) -> (337.0813, 130.6825) projected
  line L38 (337.0813, 130.6825) -> (336.8308, 130.8193) projected
  line L39 (336.8308, 130.8193) -> (336.5635, 130.919) projected
  line L40 (336.5635, 130.919) -> (336.2846, 130.9796) projected
  line L41 (336.2846, 130.9796) -> (336, 131) projected
  line L42 (336, 131) -> (0, 131) projected
  line L43 (0, 131) -> (-0.2846, 130.9796) projected
  line L44 (-0.2846, 130.9796) -> (-0.5635, 130.919) projected
  line L45 (-0.5635, 130.919) -> (-0.8308, 130.8193) projected
  line L46 (-0.8308, 130.8193) -> (-1.0813, 130.6825) projected
  line L47 (-1.0813, 130.6825) -> (-1.3097, 130.5115) projected
  line L48 (-1.3097, 130.5115) -> (-1.5115, 130.3097) projected
  line L49 (-1.5115, 130.3097) -> (-1.6825, 130.0813) projected
  line L50 (-1.6825, 130.0813) -> (-1.8193, 129.8308) projected
  line L51 (-1.8193, 129.8308) -> (-1.919, 129.5635) projected
  circle A1 centre (334.027, 128.645) radius 1.1 projected
  circle A2 centre (135.028, 128.645) radius 1.1 projected
  circle A3 centre (68.695, 128.645) radius 1.1 projected
  circle A4 centre (267.687, 2.37) radius 1.1 projected
  circle A5 centre (201.354, 2.37) radius 1.1 projected
  circle A6 centre (68.688, 2.37) radius 1.1 projected
  circle A7 centre (2.355, 2.37) radius 1.1 projected
  circle A8 centre (135.021, 2.37) radius 1.1 projected
  circle A9 centre (334.02, 2.37) radius 1.1 projected
  circle A10 centre (2.362, 128.645) radius 1.1 projected
  line L52 (4, 126) -> (332, 126) projected
  arc A11 (333, 125) -> (332, 126) centre (332, 125) ccw projected
  line L53 (333, 125) -> (333, 6) projected
  arc A12 (332, 5) -> (333, 6) centre (332, 6) ccw projected
  line L54 (332, 5) -> (4, 5) projected
  arc A13 (3, 6) -> (4, 5) centre (4, 6) ccw projected
  line L55 (3, 6) -> (3, 125) projected
  arc A14 (4, 126) -> (3, 125) centre (4, 125) ccw projected
  circle A15 centre (201.361, 128.645) radius 1.1 projected
  circle A16 centre (267.694, 128.645) radius 1.1 projected
  line L56 (150.9854, 9.2778) -> (150.9854, 0)
  line L57 (250.9222, 9.2778) -> (250.9222, 0)
  line L58 (148.4854, 5) -> (153.4854, 5)
  line L59 (153.4854, 5) -> (153.4854, 4.2)
  line L60 (153.4854, 4.2) -> (148.4854, 4.2)
  line L61 (148.4854, 4.2) -> (148.4854, 5)
  line L62 (248.4222, 5) -> (253.4222, 5)
  line L63 (253.4222, 5) -> (253.4222, 4.2)
  line L64 (253.4222, 4.2) -> (248.4222, 4.2)
  line L65 (248.4222, 4.2) -> (248.4222, 5)
  line L66 (168.1312, 122.2139) -> (180.065, 122.2139) construction
  line L67 (173.9748, 124.4692) -> (161.9748, 124.4692)
  line L68 (161.9748, 124.4692) -> (161.9748, 132.8429)
  line L69 (161.9748, 132.8429) -> (173.9748, 132.8429)
  line L70 (173.9748, 132.8429) -> (173.9748, 124.4692)
  point P0 (371.545, 162.609)
  point P1 (150.9854, 4.6389)
  point P2 (153.4854, 4.6)
  point P3 (250.9222, 4.6389)
  point P4 (253.4222, 4.6)
  point P5 (253.4222, 5)
  point P6 (153.4854, 5)
  dimension "d118" = 5
  dimension "d119" = 0.8
  dimension "d120" = 5
  dimension "d121" = 0.8
  dimension "d123" = 2.5
  dimension "d124" = 2.5
  dimension "d128" = 12
  constraints: 30 end point, 6 parallel, 5 perpendicular, 4 horizontal, 4 midpoint, 4 point on line, 2 vertical, 2 other
  measures "d118" distance of L59.end L60.end
  measures "d119" distance of L58.end L59.end
  measures "d120" distance of L63.end L64.end
  measures "d121" distance of L62.end L63.end
  measures "d123" horizontal distance of point (150.985, 4.639) point (153.485, 4.6)
  measures "d124" horizontal distance of point (250.922, 4.639) point (253.422, 4.6)
  measures "d128" distance between parallel lines of L68 L70
extrude "Extrusion4" cut sketch "Sketch9" against normal blind 10 contours L68 L69 L70 L42 | L42 L70 L52 L68 | L52 L70 L67 L68 | L60 L61 L54 L56 | L56 L54 L59 L60 | L64 L65 L54 L57 | L57 L54 L63 L64
body "Solid1"
